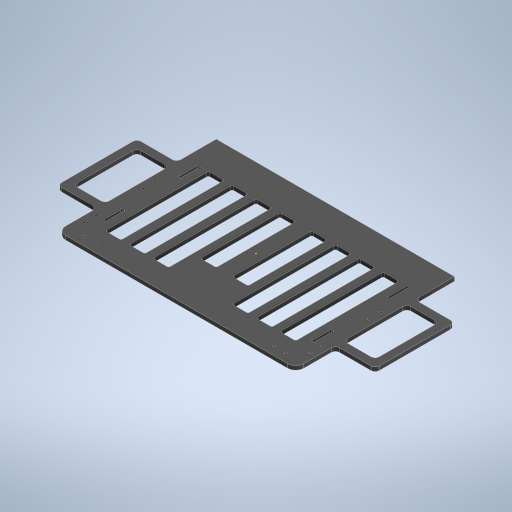
# Autodesk Inventor part: RP_Waist-Avobe
Saved by Autodesk Inventor 2024.3 (Build 283343000, 343)
## iProperties
Created: 2025-04-20
Part Number: RP_Waist-Avobe
Material: A5052
Document SubType Name: Modeling
Designer: ngt-a
Density: 2.68 g/cm^3
Appearance: 一般
Mass: 584.318 g
Surface Area: 1084.74 cm^2
Volume: 218.029 cm^3
Author: ngt-a
Autodesk Inventor part; units mm, degrees
ref_plane "YZ Plane" through (0, 0, 0) normal (1, 0, 0) x (0, 1, 0)
ref_plane "XZ Plane" through (0, 0, 0) normal (0, 1, 0) x (-1, 0, 0)
ref_plane "XY Plane" through (0, 0, 0) normal (0, 0, 1) x (1, 0, 0)
sketch "スケッチ1" plane through (0, 0, 0) normal (0, 1, 0) x (-1, 0, 0)
  line L0 (150, -95) -> (-150, -95)
  line L1 (-150, -95) -> (-150, 95)
  line L2 (-150, 95) -> (150, 95)
  line L3 (150, 95) -> (150, -95)
  line L4 (150, -95) -> (-150, 95) construction
  line L5 (-150, -95) -> (150, 95) construction
  line L6 (150, 95) -> (-150, 95)
  line L7 (-150, 95) -> (-150, 100)
  line L8 (-150, 100) -> (150, 100)
  line L9 (150, 100) -> (150, 95)
  line L10 (150, -50) -> (200, -50)
  line L11 (200, -50) -> (200, 50)
  line L12 (200, 50) -> (150, 50)
  line L13 (150, 50) -> (150, -50)
  line L14 (-150, -50) -> (-200, -50)
  line L15 (-200, -50) -> (-200, 50)
  line L16 (-200, 50) -> (-150, 50)
  line L17 (-150, 50) -> (-150, -50)
  line L18 (190, -40) -> (160, -40)
  line L19 (160, -40) -> (160, 40)
  line L20 (160, 40) -> (190, 40)
  line L21 (190, 40) -> (190, -40)
  line L22 (-190, -40) -> (-160, -40)
  line L23 (-160, -40) -> (-160, 40)
  line L24 (-160, 40) -> (-190, 40)
  line L25 (-190, 40) -> (-190, -40)
  line L26 (160, -40) -> (150, -40)
  line L27 (150, -40) -> (150, 40)
  line L28 (150, 40) -> (160, 40)
  line L29 (160, 40) -> (160, -40)
  line L30 (-160, -40) -> (-150, -40)
  line L31 (-150, -40) -> (-150, 40)
  line L32 (-150, 40) -> (-160, 40)
  line L33 (-160, 40) -> (-160, -40)
  point P0 (0, 0)
  point P1 (150, 0)
  point P2 (175, -40)
  point P3 (-155, -40)
  point P4 (-155, 40)
  point P5 (-150, 40)
  point P6 (150, 40)
  dimension "d0" = 190
  dimension "d1" = 300
  dimension "d244" = 5
  dimension "d346" = 50
  dimension "d347" = 50
  dimension "d348" = 50
  dimension "d349" = 50
  dimension "d350" = 10
  dimension "d351" = 10
  dimension "d352" = 80
  constraints: 68 end point, 16 parallel, 8 perpendicular, 6 horizontal, 6 midpoint, 6 point on line, 6 other
  measures "d0" distance of L0.end L1.end
  measures "d1" distance of L0.start L0.end
  measures "d244" distance between parallel lines of L2 L8
  measures "d346" distance between parallel lines of L13 L11
  measures "d347" distance from line of point (0, 0) L10
  measures "d348" distance from line of L12 point (150, 0)
  measures "d349" distance between parallel lines of L17 L15
  measures "d350" distance from line of L10 point (175, -40)
  measures "d351" distance between parallel lines of L14 L22
  measures "d352" distance of point (-155, -40) point (-155, 40)
extrude "押し出し1" add sketch "スケッチ1" along normal blind 5 contours L0 L1 L2 L3 | L3 L26 L18 L21 L20 L28 L12 L11 L10 | L14 L15 L16 L1 L32 L24 L25 L22 L30 | L2 L7 L8 L9
sketch "スケッチ2" plane through (0, 5, 0) normal (0, 1, 0) x (1, 0, 0)
  circle A0 centre (-142.5, -74) radius 1.6
  circle A1 centre (142.5, -74) radius 1.6
  line L0 (-150, -95) -> (150, -95) projected
  circle A2 centre (-142.5, -59) radius 1.6
  circle A3 centre (142.5, -59) radius 1.6
  circle A4 centre (-127, -89.5) radius 1.6
  line L1 (-150, 95) -> (-150, -100) projected
  circle A5 centre (-112, -89.5) radius 1.6
  line L2 (150, 95) -> (-150, 95) projected
  line L3 (0, 95) -> (0, -95)
  line L4 (-150, -2.5) -> (150, 0)
  line L5 (150, -95) -> (150, 95) projected
  circle A6 centre (127, -89.5) radius 1.6
  circle A7 centre (112, -89.5) radius 1.6
  circle A8 centre (-142.5, 15) radius 1.6
  circle A9 centre (-142.5, 0) radius 1.6
  circle A10 centre (142.5, 15) radius 1.6
  circle A11 centre (142.5, 0) radius 1.6
  point P0 (0, 0)
  dimension "d55" = 142.5
  dimension "d56" = 285
  dimension "d57" = 3.2
  dimension "d58" = 3.2
  dimension "d59" = 21
  dimension "d60" = 21
  dimension "d61" = 15
  dimension "d62" = 15
  dimension "d63" = 3.2
  dimension "d64" = 3.2
  dimension "d67" = 5.5
  dimension "d68" = 23
  dimension "d69" = 15
  dimension "d70" = 3.2
  dimension "d71" = 3.2
  dimension "d72" = 80
  dimension "d73" = 7.5
  dimension "d74" = 15
  dimension "d75" = 3.2
  dimension "d76" = 3.2
  dimension "d245" = 3.2
  constraints: 12 centre point, 4 end point, 4 midpoint, 4 symmetric about line, 4 other
  measures "d55" horizontal distance of A0.centre point (0, 0)
  measures "d56" distance of A1.centre A0.centre
  measures "d57" diameter of A0
  measures "d58" diameter of A1
  measures "d59" distance from line of L0 A0.centre
  measures "d60" distance from line of L0 A1.centre
  measures "d61" distance of A0.centre A2.centre
  measures "d62" distance of A1.centre A3.centre
  measures "d63" diameter of A3
  measures "d64" diameter of A2
  measures "d67" distance from line of L0 A4.centre
  measures "d68" distance from line of A4.centre L1
  measures "d69" distance of A5.centre A4.centre
  measures "d70" diameter of A5
  measures "d71" diameter of A4
  measures "d72" distance from line of A8.centre L2
  measures "d73" distance from line of A8.centre L1
  measures "d74" distance of A9.centre A8.centre
  measures "d75" diameter of A9
  measures "d76" diameter of A8
  measures "d245" diameter of A7
extrude "押し出し4" cut sketch "スケッチ2" against normal blind 10 contours A0 | A1 | A11 L4 | L4 A11 | A2 | A3 | A4 | A5 | A6 | A7 | A8 | A9 | A10
sketch "スケッチ4" plane through (0, 5, 0) normal (0, 1, 0) x (1, 0, 0)
  point P0 (0, 0)
sketch "スケッチ14" plane through (150, 0, -95) normal (0, 0, -1) x (-1, 0, 0)
  line L0 (0, 0) -> (300, 0) projected
  line L1 (300, 0) -> (300, 5) projected
  line L2 (0, 5) -> (300, 5) projected
  line L3 (0, 0) -> (0, 5) projected
  point P0 (150, 0)
extrude "押し出し13" add sketch "スケッチ14" along normal blind 5
fillet "フィレット3" radius 10 2 edges at (150, 2.5, 100) (-150, 2.5, 100)
sketch "スケッチ19" plane through (0, 0, 0) normal (0, -1, 0) x (1, 0, 0)
  line L0 (150, -100) -> (-150, -100) projected
  line L1 (-140, 100) -> (140, 100) projected
  line L2 (150, 90) -> (150, -100) projected
  line L3 (-150, 90) -> (-150, -100) projected
  line L4 (-120, -60) -> (120, -60)
  line L5 (120, -60) -> (120, 70)
  line L6 (120, 70) -> (-120, 70)
  line L7 (-120, 70) -> (-120, -60)
  line L8 (-120, -60) -> (-100, -60)
  line L9 (-100, -60) -> (-100, 70)
  line L10 (-100, 70) -> (-120, 70)
  line L11 (-120, 70) -> (-120, -60)
  line L12 (-90, -60) -> (-70, -60)
  line L13 (-70, -60) -> (-70, 70)
  line L14 (-70, 70) -> (-90, 70)
  line L15 (-90, 70) -> (-90, -60)
  line L16 (-60, -60) -> (-40, -60)
  line L17 (-40, -60) -> (-40, 70)
  line L18 (-40, 70) -> (-60, 70)
  line L19 (-60, 70) -> (-60, -60)
  line L20 (-30, -60) -> (-10, -60)
  line L21 (-10, -60) -> (-10, 70)
  line L22 (-10, 70) -> (-30, 70)
  line L23 (-30, 70) -> (-30, -60)
  line L24 (120, -60) -> (100, -60)
  line L25 (100, -60) -> (100, 70)
  line L26 (100, 70) -> (120, 70)
  line L27 (120, 70) -> (120, -60)
  line L28 (90, -60) -> (70, -60)
  line L29 (70, -60) -> (70, 70)
  line L30 (70, 70) -> (90, 70)
  line L31 (90, 70) -> (90, -60)
  line L32 (60, -60) -> (40, -60)
  line L33 (40, -60) -> (40, 70)
  line L34 (40, 70) -> (60, 70)
  line L35 (60, 70) -> (60, -60)
  line L36 (30, -60) -> (10, -60)
  line L37 (10, -60) -> (10, 70)
  line L38 (10, 70) -> (30, 70)
  line L39 (30, 70) -> (30, -60)
  line L40 (0, -60) -> (10, -60)
  line L41 (10, -60) -> (10, 40)
  line L42 (10, 40) -> (0, 40)
  line L43 (0, 40) -> (0, -60)
  line L44 (-10, -60) -> (0, -60)
  line L45 (0, -60) -> (0, 40)
  line L46 (0, 40) -> (-10, 40)
  line L47 (-10, 40) -> (-10, -60)
  line L48 (20, -60) -> (-20, -60)
  line L49 (-20, -60) -> (-20, 20)
  line L50 (-20, 20) -> (20, 20)
  line L51 (20, 20) -> (20, -60)
  line L52 (-30, 70) -> (-10, 70)
  line L53 (-10, 70) -> (-10, 40)
  line L54 (-10, 40) -> (-30, 40)
  line L55 (-30, 40) -> (-30, 70)
  line L56 (10, 40) -> (30, 40)
  line L57 (30, 40) -> (30, 70)
  line L58 (30, 70) -> (10, 70)
  line L59 (10, 70) -> (10, 40)
  point P0 (-5, 40)
  point P1 (-30, 70)
  point P2 (-60, 70)
  point P3 (-30, 40)
  point P4 (30, 40)
  dimension "d320" = 130
  dimension "d317" = 30
  dimension "d318" = 30
  dimension "d319" = 40
  dimension "d321" = 20
  dimension "d322" = 10
  dimension "d323" = 20
  dimension "d324" = 10
  dimension "d325" = 20
  dimension "d326" = 20
  dimension "d327" = 10
  dimension "d328" = 20
  dimension "d329" = 10
  dimension "d330" = 20
  dimension "d331" = 10
  dimension "d332" = 20
  dimension "d333" = 10
  dimension "d334" = 20
  dimension "d335" = 10
  dimension "d336" = 10
  dimension "d337" = 10
  dimension "d338" = 10
  dimension "d339" = 30
  dimension "d340" = 30
  dimension "d341" = 10
  dimension "d342" = 10
  dimension "d343" = 50
  dimension "d345" = 30
  constraints: 108 end point, 27 parallel, 13 horizontal, 13 perpendicular, 3 point on line, 1 midpoint, 1 vertical, 23 other
  measures "d317" distance between parallel lines of L2 L5
  measures "d318" distance between parallel lines of L3 L7
  measures "d321" distance between parallel lines of L7 L9
  measures "d322" distance between parallel lines of L9 L15
  measures "d323" distance between parallel lines of L15 L13
  measures "d324" distance between parallel lines of L13 L19
  measures "d325" distance between parallel lines of L19 L17
  measures "d326" distance between parallel lines of L5 L25
  measures "d327" distance between parallel lines of L17 L23
  measures "d328" distance between parallel lines of L23 L21
  measures "d329" distance between parallel lines of L25 L31
  measures "d330" distance between parallel lines of L31 L29
  measures "d331" distance between parallel lines of L29 L35
  measures "d332" distance between parallel lines of L35 L33
  measures "d333" distance between parallel lines of L39 L33
  measures "d334" distance between parallel lines of L39 L37
  measures "d335" distance between parallel lines of L41 L43
  measures "d336" distance between parallel lines of L45 L47
  measures "d337" distance between parallel lines of L37 L45
  measures "d338" distance between parallel lines of L21 L43
  measures "d341" distance between parallel lines of L47 L49
  measures "d342" distance between parallel lines of L41 L51
extrude "押し出し18" cut sketch "スケッチ19" against normal blind 5 contours L7 L6 L9 L4 | L15 L6 L13 L4 | L19 L6 L17 L4 | L23 L54 L21 L50 L49 L4 | L49 L50 L21 L4 | L37 L50 L51 L4 | L56 L39 L4 L51 L50 L37 | L6 L35 L4 L33 | L6 L31 L4 L29 | L6 L5 L4 L25
sketch "スケッチ20" plane through (0, 0, 0) normal (0, -1, 0) x (1, 0, 0)
  line L0 (133, 35.4) -> (130, 35.4)
  line L1 (130, 35.4) -> (130, 60.4)
  line L2 (130, 60.4) -> (133, 60.4)
  line L3 (133, 60.4) -> (133, 35.4)
  circle A0 centre (127, 89.5) radius 1.6 projected
  line L4 (133, -59.6) -> (130, -59.6)
  line L5 (130, -59.6) -> (130, -34.6)
  line L6 (130, -34.6) -> (133, -34.6)
  line L7 (133, -34.6) -> (133, -59.6)
  arc A1 (133, -59.6) -> (133, -57.6) centre (133, -58.6) ccw
  arc A2 (130, -57.6) -> (130, -59.6) centre (130, -58.6) ccw
  arc A3 (133, -36.6) -> (133, -34.6) centre (133, -35.6) ccw
  arc A4 (130, -34.6) -> (130, -36.6) centre (130, -35.6) ccw
  arc A5 (133, 58.4) -> (133, 60.4) centre (133, 59.4) ccw
  arc A6 (130, 60.4) -> (130, 58.4) centre (130, 59.4) ccw
  arc A7 (133, 35.4) -> (133, 37.4) centre (133, 36.4) ccw
  arc A8 (130, 37.4) -> (130, 35.4) centre (130, 36.4) ccw
  line L8 (0, 0) -> (0, 29.3825)
  line L9 (-133, 35.4) -> (-130, 35.4)
  line L10 (-130, 35.4) -> (-130, 60.4)
  line L11 (-130, 60.4) -> (-133, 60.4)
  line L12 (-133, 60.4) -> (-133, 35.4)
  line L13 (-133, -59.6) -> (-130, -59.6)
  line L14 (-130, -59.6) -> (-130, -34.6)
  line L15 (-130, -34.6) -> (-133, -34.6)
  line L16 (-133, -34.6) -> (-133, -59.6)
  arc A9 (-133, -57.6) -> (-133, -59.6) centre (-133, -58.6) ccw
  arc A10 (-130, -59.6) -> (-130, -57.6) centre (-130, -58.6) ccw
  arc A11 (-133, -34.6) -> (-133, -36.6) centre (-133, -35.6) ccw
  arc A12 (-130, -36.6) -> (-130, -34.6) centre (-130, -35.6) ccw
  arc A13 (-133, 60.4) -> (-133, 58.4) centre (-133, 59.4) ccw
  arc A14 (-130, 58.4) -> (-130, 60.4) centre (-130, 59.4) ccw
  arc A15 (-133, 37.4) -> (-133, 35.4) centre (-133, 36.4) ccw
  arc A16 (-130, 35.4) -> (-130, 37.4) centre (-130, 36.4) ccw
  point P0 (131.5, 60.4)
  point P1 (131.5, 35.4)
  point P2 (131.5, -34.6)
  point P3 (-131.5, 60.4)
  point P4 (-131.5, 35.4)
  point P5 (-131.5, -34.6)
  dimension "d272" = 3
  dimension "d273" = 4.5
  dimension "d274" = 27.5
  dimension "d275" = 25
  dimension "d276" = 25
  dimension "d277" = 70
  dimension "d278" = 3
  dimension "d279" = 3
  dimension "d280" = 1
  dimension "d281" = 1
  dimension "d282" = 1
  dimension "d283" = 1
  dimension "d284" = 1
  dimension "d285" = 1
  dimension "d286" = 1
  dimension "d287" = 1
  constraints: 34 end point, 32 point on circle, 27 symmetric about line, 16 centre point, 16 point on line, 8 tangent, 4 parallel, 3 midpoint, 2 horizontal, 2 perpendicular, 1 vertical, 8 other
  measures "d272" distance between parallel lines of L1 L3
  measures "d273" horizontal distance of A0.centre point (131.5, 60.4)
  measures "d274" distance edge to line of A0 L2
  measures "d275" distance of point (131.5, 60.4) point (131.5, 35.4)
  measures "d276" distance of L6.end L4.start
  measures "d277" distance of point (131.5, 35.4) point (131.5, -34.6)
  measures "d278" distance between parallel lines of L5 L7
  measures "d279" distance from line of A0.centre L5
  measures "d280" radius of A1
  measures "d281" radius of A2
  measures "d282" radius of A3
  measures "d283" radius of A4
  measures "d284" radius of A5
  measures "d285" radius of A6
  measures "d286" radius of A7
  measures "d287" radius of A8
extrude "押し出し19" cut sketch "スケッチ20" against normal blind 5 contours L0 L1 L2 L3 | L3 A7 | A8 L1 | L3 A5 | A6 L1 | L4 L5 L6 L7 | L7 A1 | A2 L5 | L7 A3 | A4 L5 | L12 L11 L10 L9 | A15 L12 | L10 A16 | A13 L12 | L10 A14 | L16 L15 L14 L13 | A9 L16 | L14 A10 | A11 L16 | L14 A12
fillet "フィレット11" radius 2 32 edges at (-120, 2.5, 70) (-90, 2.5, 70) (-60, 2.5, 70) (-10, 2.5, 40) (40, 2.5, 70) (70, 2.5, 70) (100, 2.5, 70) (-100, 2.5, 70) (-70, 2.5, 70) (-40, 2.5, 70) (10, 2.5, 40) (60, 2.5, 70) (90, 2.5, 70) (120, 2.5, 70) (120, 2.5, -60) (90, 2.5, -60) (60, 2.5, -60) (30, 2.5, -60) (10, 2.5, -60) (-10, 2.5, -60) (-40, 2.5, -60) (-70, 2.5, -60) (-100, 2.5, -60) (100, 2.5, -60) (70, 2.5, -60) (40, 2.5, -60) (-30, 2.5, -60) (-60, 2.5, -60) (-90, 2.5, -60) (-120, 2.5, -60) (-30, 2.5, 40) (30, 2.5, 40)
fillet "フィレット12" radius 5 16 edges at (-200, 2.5, 50) (-200, 2.5, -50) (-150, 2.5, 50) (200, 2.5, 50) (150, 2.5, 50) (150, 2.5, -40) (200, 2.5, -50) (-150, 2.5, -40) (190, 2.5, -40) (190, 2.5, 40) (-150, 2.5, 40) (-190, 2.5, 40) (150, 2.5, 40) (-190, 2.5, -40) (150, 2.5, -50) (-150, 2.5, -50)
